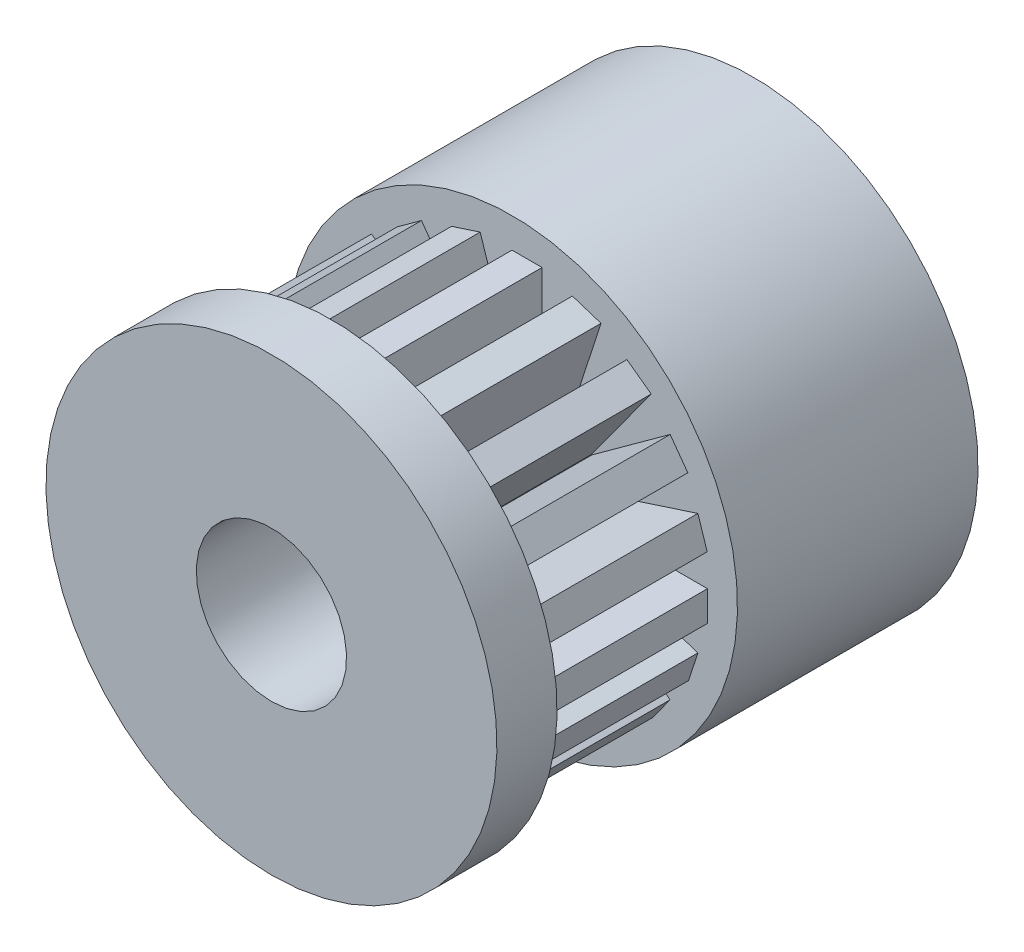
# Autodesk Inventor part: pulley20
Saved by Autodesk Inventor 2020 (Build 240168000, 168)
## iProperties
Created: 2022-12-14
Part Number: pulley20
Material: Generic
Document SubType Name: Modeling
Designer: Manish
Density: 1 g/cm^3
Appearance: Default
Author: Manish
Autodesk Inventor part; units mm, degrees
ref_plane "YZ Plane" through (0, 0, 0) normal (1, 0, 0) x (0, 1, 0)
ref_plane "XZ Plane" through (0, 0, 0) normal (0, 1, 0) x (-1, 0, 0)
ref_plane "XY Plane" through (0, 0, 0) normal (0, 0, 1) x (1, 0, 0)
sketch "Sketch2" plane through (0, 0, 0) normal (1, 0, 0) x (0, 1, 0)
  line L0 (0, 0) -> (-2.5, 0)
  line L1 (-2.5, 0) -> (-7.5, 0)
  line L2 (-7.5, 0) -> (-7.5, -2)
  line L3 (-7.5, -2) -> (-2.5, -2)
  line L4 (-2.5, -2) -> (-2.5, -8)
  line L5 (-2.5, -8) -> (-7.5, -8)
  line L6 (-7.5, -8) -> (-7.5, -16)
  line L7 (-7.5, -16) -> (-2.5, -16)
  line L8 (-2.5, -16) -> (-2.5, 0)
  line L9 (-3.284, -8) -> (-3.284, -2)
  line L10 (0, -19.2) -> (0, 3.2) projected
  point P0 (-2.5, -2)
  dimension "d1" = 2.5
  dimension "d2" = 5
  dimension "d3" = 2
  dimension "d4" = 6
  dimension "d5" = 8
  constraints: 20 end point, 6 point on line, 5 perpendicular, 1 collinear, 1 horizontal, 1 vertical
  measures "d1" distance of L0.start L0.end
  measures "d2" distance of L0.end L1.end
  measures "d3" distance of L1.end L2.end
  measures "d4" distance of L3.end L4.end
  measures "d5" distance of L5.end L6.end
revolve "Revolution1" add sketch "Sketch2" angle 360 about axis through (0, 0, -10) along (0, 0, 1)
sketch "Sketch4" plane through (0, 0, -8) normal (0, 0, 1) x (1, 0, 0)
  circle A0 centre (0, 0) radius 2.5 projected
  line L0 (0, -2.5) -> (0, -6.5)
  line L1 (0, -6.5) -> (-1, -6.5)
  line L2 (-1, -6.5) -> (-1, -2.2755)
  point P0 (-1, -2.2913)
  dimension "d14" = 4
  dimension "d15" = 1
  constraints: 6 end point, 2 perpendicular, 1 vertical, 2 other
  measures "d14" distance of L0.start L0.end
  measures "d15" distance of L0.end L1.end
extrude "Extrusion2" add sketch "Sketch4" along normal blind 6 contours L0 L1 L2 A0
pattern_circular "Circular Pattern2" count 20 over 360 about axis through (0, 0, -10) along (0, 0, 1) of "Extrusion2"
ref_plane "Work Plane1" through (0, 0, 0) normal (0, 0, 1) x (1, 0, 0)
body "Solid1"
